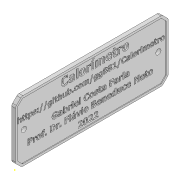
# Autodesk Inventor part: Placa
Saved by Autodesk Inventor 2020 (Build 240168000, 168)
## iProperties
Created: 2022-08-02
Part Number: Placa
Material: Genérico
Document SubType Name: Modeling
Designer: gabri
Density: 1 g/cm^3
Appearance: Padrão
Author: gabri
Autodesk Inventor part; units mm, degrees
(part 1 of 4)
ref_plane "YZ Plane" through (0, 0, 0) normal (1, 0, 0) x (0, 1, 0)
ref_plane "XZ Plane" through (0, 0, 0) normal (0, 1, 0) x (-1, 0, 0)
ref_plane "XY Plane" through (0, 0, 0) normal (0, 0, 1) x (1, 0, 0)
sketch "Esboço1" plane through (0, 0, 0) normal (1, 0, 0) x (0, 1, 0)
  line L0 (0, 0) -> (40, 0)
  line L1 (40, 0) -> (40, -100)
  line L2 (40, -100) -> (0, -100)
  line L3 (0, -100) -> (0, 0)
  dimension "d0" = 100
  dimension "d1" = 40
  constraints: 8 end point, 2 parallel, 1 horizontal, 1 perpendicular
  measures "d0" distance of L2.end L0.start
  measures "d1" distance of L1.end L2.end
extrude "Extrusão1" add sketch "Esboço1" along normal blind 2
sketch "Esboço3" plane through (2, 0, 0) normal (1, 0, 0) x (0, 0, -1)
  circle A0 centre (94, 20) radius 1.75
  circle A1 centre (6, 20) radius 1.75
  line L0 (100, 0) -> (100, 40) projected
  line L1 (0, 40) -> (0, 0) projected
  line L2 (0, 0) -> (100, 0) projected
  dimension "d4" = 3.5
  dimension "d5" = 3.5
  dimension "d6" = 6
  dimension "d7" = 6
  dimension "d10" = 40
  dimension "d11" = 20
  dimension "d12" = 20
  constraints: 2 centre point
  measures "d4" diameter of A0
  measures "d5" diameter of A1
  measures "d6" distance from line of L0 A0.centre
  measures "d7" distance from line of L1 A1.centre
  measures "d10" distance of L1.start L1.end
  measures "d11" distance from line of L2 A1.centre
  measures "d12" distance from line of L2 A0.centre
extrude "Extrusão2" cut sketch "Esboço3" against normal blind 4
sketch "Esboço2" plane through (2, 0, 0) normal (1, 0, 0) x (0, 0, -1)
  line L0 (30.0469, 37.5277) -> (51.3829, 37.5277) construction
  line L1 (51.3829, 37.5277) -> (51.3829, 32.8173) construction
  line L2 (51.3829, 32.8173) -> (30.0469, 32.8173) construction
  line L3 (30.0469, 32.8173) -> (30.0469, 37.5277) construction
  line L4 (1.6337, 28.6211) -> (100.4753, 28.6211) construction
  line L5 (100.4753, 28.6211) -> (100.4753, 23.9424) construction
  line L6 (100.4753, 23.9424) -> (1.6337, 23.9424) construction
  line L7 (1.6337, 23.9424) -> (1.6337, 28.6211) construction
  line L8 (1.8628, 19.959) -> (97.4553, 19.959) construction
  line L9 (97.4553, 19.959) -> (97.4553, 12.3141) construction
  line L10 (97.4553, 12.3141) -> (1.8628, 12.3141) construction
  line L11 (1.8628, 12.3141) -> (1.8628, 19.959) construction
  line L12 (1.4175, 13.8251) -> (97.3864, 13.8251) construction
  line L13 (97.3864, 13.8251) -> (97.3864, 4.9391) construction
  line L14 (97.3864, 4.9391) -> (1.4175, 4.9391) construction
  line L15 (1.4175, 4.9391) -> (1.4175, 13.8251) construction
  line L16 (0.4004, 6.6404) -> (95.5795, 6.6404) construction
  line L17 (95.5795, 6.6404) -> (95.5795, -2.443) construction
  line L18 (95.5795, -2.443) -> (0.4004, -2.443) construction
  line L19 (0.4004, -2.443) -> (0.4004, 6.6404) construction
  spline S0 degree 2 poles (32.9886, 31.2299) (31.7495, 31.2299) (30.2965, 32.7275) (30.2965, 34.0824) knots 0 0 0 1 2 2 2
  spline S1 degree 2 poles (30.2965, 34.0824) (30.2965, 35.3883) (31.7539, 36.9438) (32.993, 36.9438) knots 0 0 0 1 2 2 2
  spline S2 degree 2 poles (32.993, 36.9438) (33.3184, 36.9438) (33.8443, 36.8681) (34.085, 36.8057) knots 0 0 0 1 2 2 2
  spline S3 degree 2 poles (34.085, 36.8057) (34.2722, 36.7477) (34.7134, 36.5561) (34.8516, 36.4848) knots 0 0 0 1 2 2 2
  line L20 (34.8516, 36.4848) -> (34.8516, 35.1744)
  line L21 (34.8516, 35.1744) -> (34.7134, 35.1744)
  spline S4 degree 2 poles (34.7134, 35.1744) (34.6109, 35.2635) (34.3078, 35.5131) (34.1162, 35.629) knots 0 0 0 1 2 2 2
  spline S5 degree 2 poles (34.1162, 35.629) (33.9245, 35.7493) (33.4655, 35.9143) (33.2114, 35.9143) knots 0 0 0 1 2 2 2
  spline S6 degree 2 poles (33.2114, 35.9143) (32.9128, 35.9143) (32.418, 35.7271) (32.1907, 35.4908) knots 0 0 0 1 2 2 2
  spline S7 degree 2 poles (32.1907, 35.4908) (31.9857, 35.2814) (31.7227, 34.5638) (31.7227, 34.078) knots 0 0 0 1 2 2 2
  spline S8 degree 2 poles (31.7227, 34.078) (31.7227, 33.5654) (31.9946, 32.8656) (32.2175, 32.6517) knots 0 0 0 1 2 2 2
  spline S9 degree 2 poles (32.2175, 32.6517) (32.4314, 32.4422) (32.9574, 32.2595) (33.2203, 32.2595) knots 0 0 0 1 2 2 2
  spline S10 degree 2 poles (33.2203, 32.2595) (33.4922, 32.2595) (33.9869, 32.4422) (34.1563, 32.5536) knots 0 0 0 1 2 2 2
  spline S11 degree 2 poles (34.1563, 32.5536) (34.3435, 32.6651) (34.6243, 32.9013) (34.7268, 32.9949) knots 0 0 0 1 2 2 2
  line L22 (34.7268, 32.9949) -> (34.8516, 32.9949)
  line L23 (34.8516, 32.9949) -> (34.8516, 31.7023)
  spline S12 degree 2 poles (34.8516, 31.7023) (34.7001, 31.631) (34.3034, 31.4528) (34.0894, 31.3904) knots 0 0 0 1 2 2 2
  spline S13 degree 2 poles (34.0894, 31.3904) (33.8309, 31.3101) (33.3808, 31.2299) (32.9886, 31.2299) knots 0 0 0 1 2 2 2
  spline S14 degree 2 poles (37.8779, 31.7781) (37.7442, 31.6667) (37.5347, 31.4884) (37.3565, 31.3993) knots 0 0 0 1 2 2 2
  spline S15 degree 2 poles (37.3565, 31.3993) (37.1826, 31.3146) (36.8528, 31.2254) (36.5586, 31.2254) knots 0 0 0 1 2 2 2
  spline S16 degree 2 poles (36.5586, 31.2254) (36.006, 31.2254) (35.2795, 31.9653) (35.2795, 32.5269) knots 0 0 0 1 2 2 2
  spline S17 degree 2 poles (35.2795, 32.5269) (35.2795, 32.986) (35.6494, 33.5565) (35.9971, 33.7214) knots 0 0 0 1 2 2 2
  spline S18 degree 2 poles (35.9971, 33.7214) (36.3492, 33.8908) (37.3253, 34.0245) (37.8869, 34.0601) knots 0 0 0 1 2 2 2
  line L24 (37.8869, 34.0601) -> (37.8869, 34.0824)
  spline S19 degree 2 poles (37.8869, 34.0824) (37.8869, 34.4256) (37.3787, 34.6886) (36.8706, 34.6886) knots 0 0 0 1 2 2 2
  spline S20 degree 2 poles (36.8706, 34.6886) (36.6433, 34.6886) (36.0283, 34.5237) (35.7386, 34.3944) knots 0 0 0 1 2 2 2
  line L25 (35.7386, 34.3944) -> (35.6271, 34.3944)
  line L26 (35.6271, 34.3944) -> (35.6271, 35.3972)
  spline S21 degree 2 poles (35.6271, 35.3972) (35.8188, 35.4507) (36.6745, 35.6023) (37.1113, 35.6023) knots 0 0 0 1 2 2 2
  spline S22 degree 2 poles (37.1113, 35.6023) (38.181, 35.6023) (39.1616, 34.8891) (39.1616, 34.1582) knots 0 0 0 1 2 2 2
  line L27 (39.1616, 34.1582) -> (39.1616, 31.3369)
  line L28 (39.1616, 31.3369) -> (37.8779, 31.3369)
  line L29 (37.8779, 31.3369) -> (37.8779, 31.7781)
  line L30 (37.8779, 32.4199) -> (37.8779, 33.2801)
  spline S23 degree 2 poles (37.8779, 33.2801) (37.5481, 33.2489) (37.1425, 33.1999) (36.9464, 33.1286) knots 0 0 0 1 2 2 2
  spline S24 degree 2 poles (36.9464, 33.1286) (36.7726, 33.0707) (36.5854, 32.83) (36.5854, 32.6339) knots 0 0 0 1 2 2 2
  spline S25 degree 2 poles (36.5854, 32.6339) (36.5854, 32.3442) (36.9018, 32.1258) (37.2094, 32.1258) knots 0 0 0 1 2 2 2
  spline S26 degree 2 poles (37.2094, 32.1258) (37.3787, 32.1258) (37.7353, 32.2818) (37.8779, 32.4199) knots 0 0 0 1 2 2 2
  line L31 (41.4124, 31.3369) -> (40.1198, 31.3369)
  line L32 (40.1198, 31.3369) -> (40.1198, 37.082)
  line L33 (40.1198, 37.082) -> (41.4124, 37.082)
  line L34 (41.4124, 37.082) -> (41.4124, 31.3369)
  spline S27 degree 2 poles (46.382, 33.4094) (46.382, 32.3843) (45.2633, 31.2076) (44.2426, 31.2076) knots 0 0 0 1 2 2 2
  spline S28 degree 2 poles (44.2426, 31.2076) (43.2264, 31.2076) (42.0988, 32.3843) (42.0988, 33.4094) knots 0 0 0 1 2 2 2
  spline S29 degree 2 poles (42.0988, 33.4094) (42.0988, 34.4434) (43.2264, 35.6156) (44.2426, 35.6156) knots 0 0 0 1 2 2 2
  spline S30 degree 2 poles (44.2426, 35.6156) (45.2588, 35.6156) (46.382, 34.439) (46.382, 33.4094) knots 0 0 0 1 2 2 2
  spline S31 degree 2 poles (45.0582, 33.4005) (45.0582, 33.7704) (44.9379, 34.2651) (44.8309, 34.4122) knots 0 0 0 1 2 2 2
  spline S32 degree 2 poles (44.8309, 34.4122) (44.7151, 34.5682) (44.4253, 34.6886) (44.2426, 34.6886) knots 0 0 0 1 2 2 2
  spline S33 degree 2 poles (44.2426, 34.6886) (44.0643, 34.6886) (43.7835, 34.5816) (43.6676, 34.4301) knots 0 0 0 1 2 2 2
  spline S34 degree 2 poles (43.6676, 34.4301) (43.5562, 34.2874) (43.4225, 33.7838) (43.4225, 33.4005) knots 0 0 0 1 2 2 2
  spline S35 degree 2 poles (43.4225, 33.4005) (43.4225, 33.0216) (43.5473, 32.5536) (43.6498, 32.411) knots 0 0 0 1 2 2 2
  spline S36 degree 2 poles (43.6498, 32.411) (43.7523, 32.2684) (44.0643, 32.1347) (44.2515, 32.1347) knots 0 0 0 1 2 2 2
  spline S37 degree 2 poles (44.2515, 32.1347) (44.4075, 32.1347) (44.7284, 32.2684) (44.8265, 32.4021) knots 0 0 0 1 2 2 2
  spline S38 degree 2 poles (44.8265, 32.4021) (44.9379, 32.5581) (45.0582, 33.0083) (45.0582, 33.4005) knots 0 0 0 1 2 2 2
  line L35 (49.854, 34.2607) -> (49.7471, 34.2607)
  spline S39 degree 2 poles (49.7471, 34.2607) (49.6713, 34.2874) (49.3905, 34.3142) (49.2211, 34.3142) knots 0 0 0 1 2 2 2
  spline S40 degree 2 poles (49.2211, 34.3142) (49.0206, 34.3142) (48.5704, 34.1938) (48.3609, 34.1136) knots 0 0 0 1 2 2 2
  line L36 (48.3609, 34.1136) -> (48.3609, 31.3369)
  line L37 (48.3609, 31.3369) -> (47.0684, 31.3369)
  line L38 (47.0684, 31.3369) -> (47.0684, 35.4864)
  line L39 (47.0684, 35.4864) -> (48.3609, 35.4864)
  line L40 (48.3609, 35.4864) -> (48.3609, 34.8891)
  spline S41 degree 2 poles (48.3609, 34.8891) (48.4501, 34.9694) (48.7621, 35.219) (48.8913, 35.2947) knots 0 0 0 1 2 2 2
  spline S42 degree 2 poles (48.8913, 35.2947) (49.0339, 35.3794) (49.4083, 35.4998) (49.5732, 35.4998) knots 0 0 0 1 2 2 2
  spline S43 degree 2 poles (49.5732, 35.4998) (49.6356, 35.4998) (49.7916, 35.4908) (49.854, 35.4864) knots 0 0 0 1 2 2 2
  line L41 (49.854, 35.4864) -> (49.854, 34.2607)
  line L42 (51.6413, 31.3369) -> (50.3488, 31.3369)
  line L43 (50.3488, 31.3369) -> (50.3488, 35.4864)
  line L44 (50.3488, 35.4864) -> (51.6413, 35.4864)
  line L45 (51.6413, 35.4864) -> (51.6413, 31.3369)
  line L46 (52.194, 37.5277) -> (51.0842, 36.0747)
  line L47 (51.0842, 36.0747) -> (50.2061, 36.0747)
  line L48 (50.2061, 36.0747) -> (50.9728, 37.5277)
  line L49 (50.9728, 37.5277) -> (52.194, 37.5277)
  line L50 (57.5826, 31.3369) -> (57.5826, 33.4094)
  spline S44 degree 2 poles (57.5826, 33.4094) (57.5826, 33.7169) (57.5603, 34.1359) (57.5068, 34.2696) knots 0 0 0 1 2 2 2
  spline S45 degree 2 poles (57.5068, 34.2696) (57.4488, 34.4033) (57.2171, 34.5237) (57.0076, 34.5237) knots 0 0 0 1 2 2 2
  spline S46 degree 2 poles (57.0076, 34.5237) (56.8605, 34.5237) (56.5753, 34.3944) (56.4059, 34.2741) knots 0 0 0 1 2 2 2
  line L51 (56.4059, 34.2741) -> (56.4059, 31.3369)
  line L52 (56.4059, 31.3369) -> (55.1044, 31.3369)
  line L53 (55.1044, 31.3369) -> (55.1044, 33.4094)
  spline S47 degree 2 poles (55.1044, 33.4094) (55.1044, 33.7125) (55.0777, 34.1359) (55.0242, 34.2696) knots 0 0 0 1 2 2 2
  spline S48 degree 2 poles (55.0242, 34.2696) (54.9663, 34.4033) (54.7345, 34.5237) (54.525, 34.5237) knots 0 0 0 1 2 2 2
  spline S49 degree 2 poles (54.525, 34.5237) (54.369, 34.5237) (54.0615, 34.3766) (53.9189, 34.2741) knots 0 0 0 1 2 2 2
  line L54 (53.9189, 34.2741) -> (53.9189, 31.3369)
  line L55 (53.9189, 31.3369) -> (52.6263, 31.3369)
  line L56 (52.6263, 31.3369) -> (52.6263, 35.4864)
  line L57 (52.6263, 35.4864) -> (53.9189, 35.4864)
  line L58 (53.9189, 35.4864) -> (53.9189, 35.0273)
  spline S50 degree 2 poles (53.9189, 35.0273) (54.2353, 35.2947) (54.8014, 35.5978) (55.1535, 35.5978) knots 0 0 0 1 2 2 2
  spline S51 degree 2 poles (55.1535, 35.5978) (55.5323, 35.5978) (56.1117, 35.2368) (56.2633, 34.8758) knots 0 0 0 1 2 2 2
  spline S52 degree 2 poles (56.2633, 34.8758) (56.6332, 35.2234) (57.2928, 35.5978) (57.6316, 35.5978) knots 0 0 0 1 2 2 2
  spline S53 degree 2 poles (57.6316, 35.5978) (57.9213, 35.5978) (58.3804, 35.4151) (58.5364, 35.2279) knots 0 0 0 1 2 2 2
  spline S54 degree 2 poles (58.5364, 35.2279) (58.7102, 35.0273) (58.884, 34.4791) (58.884, 34.0378) knots 0 0 0 1 2 2 2
  line L59 (58.884, 34.0378) -> (58.884, 31.3369)
  line L60 (58.884, 31.3369) -> (57.5826, 31.3369)
  spline S55 degree 2 poles (61.9683, 31.2254) (60.7916, 31.2254) (59.5392, 32.3486) (59.5392, 33.3871) knots 0 0 0 1 2 2 2
  spline S56 degree 2 poles (59.5392, 33.3871) (59.5392, 34.4033) (60.7069, 35.6156) (61.7588, 35.6156) knots 0 0 0 1 2 2 2
  spline S57 degree 2 poles (61.7588, 35.6156) (62.7082, 35.6156) (63.6709, 34.5861) (63.6709, 33.6322) knots 0 0 0 1 2 2 2
  line L61 (63.6709, 33.6322) -> (63.6709, 33.1643)
  line L62 (63.6709, 33.1643) -> (60.8317, 33.1643)
  spline S58 degree 2 poles (60.8317, 33.1643) (60.8496, 32.8745) (61.0591, 32.4912) (61.2284, 32.3754) knots 0 0 0 1 2 2 2
  spline S59 degree 2 poles (61.2284, 32.3754) (61.3933, 32.2595) (61.839, 32.1614) (62.102, 32.1614) knots 0 0 0 1 2 2 2
  spline S60 degree 2 poles (62.102, 32.1614) (62.3249, 32.1614) (62.7616, 32.2595) (62.9444, 32.3442) knots 0 0 0 1 2 2 2
  spline S61 degree 2 poles (62.9444, 32.3442) (63.1048, 32.411) (63.3723, 32.5759) (63.4569, 32.6383) knots 0 0 0 1 2 2 2
  line L63 (63.4569, 32.6383) -> (63.5951, 32.6383)
  line L64 (63.5951, 32.6383) -> (63.5951, 31.5686)
  spline S62 degree 2 poles (63.5951, 31.5686) (63.4347, 31.5062) (63.1762, 31.3993) (62.9444, 31.3458) knots 0 0 0 1 2 2 2
  spline S63 degree 2 poles (62.9444, 31.3458) (62.7349, 31.2878) (62.2892, 31.2254) (61.9683, 31.2254) knots 0 0 0 1 2 2 2
  spline S64 degree 2 poles (62.3962, 33.9442) (62.3873, 34.3543) (62.0262, 34.7866) (61.6563, 34.7866) knots 0 0 0 1 2 2 2
  spline S65 degree 2 poles (61.6563, 34.7866) (61.2775, 34.7866) (60.8496, 34.332) (60.8273, 33.9442) knots 0 0 0 1 2 2 2
  line L65 (60.8273, 33.9442) -> (62.3962, 33.9442)
  spline S66 degree 2 poles (65.9217, 31.2566) (65.1328, 31.2566) (64.4108, 31.9074) (64.4108, 32.6472) knots 0 0 0 1 2 2 2
  line L66 (64.4108, 32.6472) -> (64.4108, 34.5861)
  line L67 (64.4108, 34.5861) -> (63.916, 34.5861)
  line L68 (63.916, 34.5861) -> (63.916, 35.4864)
  line L69 (63.916, 35.4864) -> (64.4108, 35.4864)
  line L70 (64.4108, 35.4864) -> (64.4108, 36.672)
  line L71 (64.4108, 36.672) -> (65.7033, 36.672)
  line L72 (65.7033, 36.672) -> (65.7033, 35.4864)
  line L73 (65.7033, 35.4864) -> (66.9513, 35.4864)
  line L74 (66.9513, 35.4864) -> (66.9513, 34.5861)
  line L75 (66.9513, 34.5861) -> (65.7033, 34.5861)
  line L76 (65.7033, 34.5861) -> (65.7033, 33.1108)
  spline S67 degree 2 poles (65.7033, 33.1108) (65.7033, 32.8924) (65.7122, 32.567) (65.7657, 32.4378) knots 0 0 0 1 2 2 2
  spline S68 degree 2 poles (65.7657, 32.4378) (65.8192, 32.3085) (66.0822, 32.157) (66.3317, 32.157) knots 0 0 0 1 2 2 2
  spline S69 degree 2 poles (66.3317, 32.157) (66.4387, 32.157) (66.773, 32.2461) (66.8398, 32.2818) knots 0 0 0 1 2 2 2
  line L77 (66.8398, 32.2818) -> (66.9513, 32.2818)
  line L78 (66.9513, 32.2818) -> (66.9513, 31.3725)
  spline S70 degree 2 poles (66.9513, 31.3725) (66.7418, 31.319) (66.2693, 31.2566) (65.9217, 31.2566) knots 0 0 0 1 2 2 2
  line L79 (70.2629, 34.2607) -> (70.1559, 34.2607)
  spline S71 degree 2 poles (70.1559, 34.2607) (70.0801, 34.2874) (69.7993, 34.3142) (69.63, 34.3142) knots 0 0 0 1 2 2 2
  spline S72 degree 2 poles (69.63, 34.3142) (69.4294, 34.3142) (68.9792, 34.1938) (68.7698, 34.1136) knots 0 0 0 1 2 2 2
  line L80 (68.7698, 34.1136) -> (68.7698, 31.3369)
  line L81 (68.7698, 31.3369) -> (67.4772, 31.3369)
  line L82 (67.4772, 31.3369) -> (67.4772, 35.4864)
  line L83 (67.4772, 35.4864) -> (68.7698, 35.4864)
  line L84 (68.7698, 35.4864) -> (68.7698, 34.8891)
  spline S73 degree 2 poles (68.7698, 34.8891) (68.8589, 34.9694) (69.1709, 35.219) (69.3001, 35.2947) knots 0 0 0 1 2 2 2
  spline S74 degree 2 poles (69.3001, 35.2947) (69.4428, 35.3794) (69.8172, 35.4998) (69.9821, 35.4998) knots 0 0 0 1 2 2 2
  spline S75 degree 2 poles (69.9821, 35.4998) (70.0445, 35.4998) (70.2005, 35.4908) (70.2629, 35.4864) knots 0 0 0 1 2 2 2
  line L85 (70.2629, 35.4864) -> (70.2629, 34.2607)
  spline S76 degree 2 poles (74.7377, 33.4094) (74.7377, 32.3843) (73.619, 31.2076) (72.5984, 31.2076) knots 0 0 0 1 2 2 2
  spline S77 degree 2 poles (72.5984, 31.2076) (71.5822, 31.2076) (70.4545, 32.3843) (70.4545, 33.4094) knots 0 0 0 1 2 2 2
  spline S78 degree 2 poles (70.4545, 33.4094) (70.4545, 34.4434) (71.5822, 35.6156) (72.5984, 35.6156) knots 0 0 0 1 2 2 2
  spline S79 degree 2 poles (72.5984, 35.6156) (73.6146, 35.6156) (74.7377, 34.439) (74.7377, 33.4094) knots 0 0 0 1 2 2 2
  spline S80 degree 2 poles (73.414, 33.4005) (73.414, 33.7704) (73.2937, 34.2651) (73.1867, 34.4122) knots 0 0 0 1 2 2 2
  spline S81 degree 2 poles (73.1867, 34.4122) (73.0708, 34.5682) (72.7811, 34.6886) (72.5984, 34.6886) knots 0 0 0 1 2 2 2
  spline S82 degree 2 poles (72.5984, 34.6886) (72.4201, 34.6886) (72.1393, 34.5816) (72.0234, 34.4301) knots 0 0 0 1 2 2 2
  spline S83 degree 2 poles (72.0234, 34.4301) (71.912, 34.2874) (71.7783, 33.7838) (71.7783, 33.4005) knots 0 0 0 1 2 2 2
  spline S84 degree 2 poles (71.7783, 33.4005) (71.7783, 33.0216) (71.9031, 32.5536) (72.0056, 32.411) knots 0 0 0 1 2 2 2
  spline S85 degree 2 poles (72.0056, 32.411) (72.1081, 32.2684) (72.4201, 32.1347) (72.6073, 32.1347) knots 0 0 0 1 2 2 2
  spline S86 degree 2 poles (72.6073, 32.1347) (72.7633, 32.1347) (73.0842, 32.2684) (73.1822, 32.4021) knots 0 0 0 1 2 2 2
  spline S87 degree 2 poles (73.1822, 32.4021) (73.2937, 32.5581) (73.414, 33.0083) (73.414, 33.4005) knots 0 0 0 1 2 2 2
  line L86 (4.4189, 24.9623) -> (3.5907, 24.9623)
  line L87 (3.5907, 24.9623) -> (3.5907, 26.2698)
  spline S88 degree 2 poles (3.5907, 26.2698) (3.5907, 26.4315) (3.5652, 26.7491) (3.5312, 26.8229) knots 0 0 0 1 2 2 2
  spline S89 degree 2 poles (3.5312, 26.8229) (3.4886, 26.9136) (3.3298, 26.9902) (3.1936, 26.9902) knots 0 0 0 1 2 2 2
  spline S90 degree 2 poles (3.1936, 26.9902) (3.0944, 26.9902) (2.8873, 26.9136) (2.771, 26.8314) knots 0 0 0 1 2 2 2
  line L88 (2.771, 26.8314) -> (2.771, 24.9623)
  line L89 (2.771, 24.9623) -> (1.9485, 24.9623)
  line L90 (1.9485, 24.9623) -> (1.9485, 28.6183)
  line L91 (1.9485, 28.6183) -> (2.771, 28.6183)
  line L92 (2.771, 28.6183) -> (2.771, 27.3107)
  spline S91 degree 2 poles (2.771, 27.3107) (2.9724, 27.4809) (3.3553, 27.6738) (3.5879, 27.6738) knots 0 0 0 1 2 2 2
  spline S92 degree 2 poles (3.5879, 27.6738) (3.9906, 27.6738) (4.4189, 27.1632) (4.4189, 26.6811) knots 0 0 0 1 2 2 2
  line L93 (4.4189, 26.6811) -> (4.4189, 24.9623)
  spline S93 degree 2 poles (6.0385, 24.9112) (5.5364, 24.9112) (5.0769, 25.3253) (5.0769, 25.7961) knots 0 0 0 1 2 2 2
  line L94 (5.0769, 25.7961) -> (5.0769, 27.0299)
  line L95 (5.0769, 27.0299) -> (4.7621, 27.0299)
  line L96 (4.7621, 27.0299) -> (4.7621, 27.6029)
  line L97 (4.7621, 27.6029) -> (5.0769, 27.6029)
  line L98 (5.0769, 27.6029) -> (5.0769, 28.3573)
  line L99 (5.0769, 28.3573) -> (5.8995, 28.3573)
  line L100 (5.8995, 28.3573) -> (5.8995, 27.6029)
  line L101 (5.8995, 27.6029) -> (6.6936, 27.6029)
  line L102 (6.6936, 27.6029) -> (6.6936, 27.0299)
  line L103 (6.6936, 27.0299) -> (5.8995, 27.0299)
  line L104 (5.8995, 27.0299) -> (5.8995, 26.0911)
  spline S94 degree 2 poles (5.8995, 26.0911) (5.8995, 25.9521) (5.9051, 25.7451) (5.9392, 25.6628) knots 0 0 0 1 2 2 2
  spline S95 degree 2 poles (5.9392, 25.6628) (5.9732, 25.5806) (6.1406, 25.4841) (6.2994, 25.4841) knots 0 0 0 1 2 2 2
  spline S96 degree 2 poles (6.2994, 25.4841) (6.3675, 25.4841) (6.5802, 25.5409) (6.6227, 25.5636) knots 0 0 0 1 2 2 2
  line L105 (6.6227, 25.5636) -> (6.6936, 25.5636)
  line L106 (6.6936, 25.5636) -> (6.6936, 24.985)
  spline S97 degree 2 poles (6.6936, 24.985) (6.5603, 24.9509) (6.2597, 24.9112) (6.0385, 24.9112) knots 0 0 0 1 2 2 2
  spline S98 degree 2 poles (8.0381, 24.9112) (7.536, 24.9112) (7.0765, 25.3253) (7.0765, 25.7961) knots 0 0 0 1 2 2 2
  line L107 (7.0765, 25.7961) -> (7.0765, 27.0299)
  line L108 (7.0765, 27.0299) -> (6.7617, 27.0299)
  line L109 (6.7617, 27.0299) -> (6.7617, 27.6029)
  line L110 (6.7617, 27.6029) -> (7.0765, 27.6029)
  line L111 (7.0765, 27.6029) -> (7.0765, 28.3573)
  line L112 (7.0765, 28.3573) -> (7.8991, 28.3573)
  line L113 (7.8991, 28.3573) -> (7.8991, 27.6029)
  line L114 (7.8991, 27.6029) -> (8.6932, 27.6029)
  line L115 (8.6932, 27.6029) -> (8.6932, 27.0299)
  line L116 (8.6932, 27.0299) -> (7.8991, 27.0299)
  line L117 (7.8991, 27.0299) -> (7.8991, 26.0911)
  spline S99 degree 2 poles (7.8991, 26.0911) (7.8991, 25.9521) (7.9047, 25.7451) (7.9388, 25.6628) knots 0 0 0 1 2 2 2
  spline S100 degree 2 poles (7.9388, 25.6628) (7.9728, 25.5806) (8.1402, 25.4841) (8.299, 25.4841) knots 0 0 0 1 2 2 2
  spline S101 degree 2 poles (8.299, 25.4841) (8.3671, 25.4841) (8.5798, 25.5409) (8.6223, 25.5636) knots 0 0 0 1 2 2 2
  line L118 (8.6223, 25.5636) -> (8.6932, 25.5636)
  line L119 (8.6932, 25.5636) -> (8.6932, 24.985)
  spline S102 degree 2 poles (8.6932, 24.985) (8.5599, 24.9509) (8.2593, 24.9112) (8.0381, 24.9112) knots 0 0 0 1 2 2 2
  spline S103 degree 2 poles (11.6146, 26.318) (11.6146, 25.6855) (10.9736, 24.9112) (10.5028, 24.9112) knots 0 0 0 1 2 2 2
  spline S104 degree 2 poles (10.5028, 24.9112) (10.3071, 24.9112) (10.015, 24.9991) (9.8504, 25.0956) knots 0 0 0 1 2 2 2
  line L120 (9.8504, 25.0956) -> (9.8504, 23.9951)
  line L121 (9.8504, 23.9951) -> (9.0279, 23.9951)
  line L122 (9.0279, 23.9951) -> (9.0279, 27.6029)
  line L123 (9.0279, 27.6029) -> (9.8504, 27.6029)
  line L124 (9.8504, 27.6029) -> (9.8504, 27.3249)
  spline S105 degree 2 poles (9.8504, 27.3249) (10.032, 27.4809) (10.4064, 27.6738) (10.6531, 27.6738) knots 0 0 0 1 2 2 2
  spline S106 degree 2 poles (10.6531, 27.6738) (11.1126, 27.6738) (11.6146, 26.9448) (11.6146, 26.318) knots 0 0 0 1 2 2 2
  spline S107 degree 2 poles (10.7722, 26.301) (10.7722, 26.6867) (10.534, 27.0328) (10.2844, 27.0328) knots 0 0 0 1 2 2 2
  spline S108 degree 2 poles (10.2844, 27.0328) (10.1738, 27.0328) (9.9554, 26.9619) (9.8504, 26.8909) knots 0 0 0 1 2 2 2
  line L125 (9.8504, 26.8909) -> (9.8504, 25.5664)
  spline S109 degree 2 poles (9.8504, 25.5664) (9.9157, 25.538) (10.0745, 25.5153) (10.1823, 25.5153) knots 0 0 0 1 2 2 2
  spline S110 degree 2 poles (10.1823, 25.5153) (10.4801, 25.5153) (10.7722, 25.9068) (10.7722, 26.301) knots 0 0 0 1 2 2 2
  spline S111 degree 2 poles (12.8598, 24.8914) (12.5705, 24.8914) (12.0514, 25.019) (11.8812, 25.1041) knots 0 0 0 1 2 2 2
  line L126 (11.8812, 25.1041) -> (11.8812, 25.799)
  line L127 (11.8812, 25.799) -> (11.9493, 25.799)
  spline S112 degree 2 poles (11.9493, 25.799) (12.0089, 25.7536) (12.1592, 25.6458) (12.2925, 25.5862) knots 0 0 0 1 2 2 2
  spline S113 degree 2 poles (12.2925, 25.5862) (12.4088, 25.5324) (12.6953, 25.4558) (12.8654, 25.4558) knots 0 0 0 1 2 2 2
  spline S114 degree 2 poles (12.8654, 25.4558) (13.0385, 25.4558) (13.3051, 25.5636) (13.3051, 25.6798) knots 0 0 0 1 2 2 2
  spline S115 degree 2 poles (13.3051, 25.6798) (13.3051, 25.7706) (13.1831, 25.867) (13.0073, 25.9068) knots 0 0 0 1 2 2 2
  spline S116 degree 2 poles (13.0073, 25.9068) (12.9137, 25.9323) (12.6272, 25.9862) (12.5166, 26.0202) knots 0 0 0 1 2 2 2
  spline S117 degree 2 poles (12.5166, 26.0202) (12.2046, 26.1166) (11.8926, 26.4939) (11.8926, 26.803) knots 0 0 0 1 2 2 2
  spline S118 degree 2 poles (11.8926, 26.803) (11.8926, 26.9789) (12.0543, 27.2909) (12.2131, 27.4128) knots 0 0 0 1 2 2 2
  spline S119 degree 2 poles (12.2131, 27.4128) (12.3691, 27.532) (12.8314, 27.6738) (13.1235, 27.6738) knots 0 0 0 1 2 2 2
  spline S120 degree 2 poles (13.1235, 27.6738) (13.4015, 27.6738) (13.8667, 27.5632) (14.0255, 27.4866) knots 0 0 0 1 2 2 2
  line L128 (14.0255, 27.4866) -> (14.0255, 26.8172)
  line L129 (14.0255, 26.8172) -> (13.9603, 26.8172)
  spline S121 degree 2 poles (13.9603, 26.8172) (13.9177, 26.8512) (13.7334, 26.9619) (13.6483, 27.0016) knots 0 0 0 1 2 2 2
  spline S122 degree 2 poles (13.6483, 27.0016) (13.5433, 27.0469) (13.2881, 27.1093) (13.1547, 27.1093) knots 0 0 0 1 2 2 2
  spline S123 degree 2 poles (13.1547, 27.1093) (12.9761, 27.1093) (12.7293, 26.9874) (12.7293, 26.8881) knots 0 0 0 1 2 2 2
  spline S124 degree 2 poles (12.7293, 26.8881) (12.7293, 26.7974) (12.8513, 26.6952) (13.0555, 26.6442) knots 0 0 0 1 2 2 2
  spline S125 degree 2 poles (13.0555, 26.6442) (13.1604, 26.6187) (13.4355, 26.5704) (13.5632, 26.5279) knots 0 0 0 1 2 2 2
  spline S126 degree 2 poles (13.5632, 26.5279) (13.8468, 26.4371) (14.1418, 26.0826) (14.1418, 25.7876) knots 0 0 0 1 2 2 2
  spline S127 degree 2 poles (14.1418, 25.7876) (14.1418, 25.6033) (13.9688, 25.2657) (13.8071, 25.1523) knots 0 0 0 1 2 2 2
  spline S128 degree 2 poles (13.8071, 25.1523) (13.6398, 25.0275) (13.1803, 24.8914) (12.8598, 24.8914) knots 0 0 0 1 2 2 2
  line L130 (15.5089, 24.9623) -> (14.6778, 24.9623)
  line L131 (14.6778, 24.9623) -> (14.6778, 25.8869)
  line L132 (14.6778, 25.8869) -> (15.5089, 25.8869)
  line L133 (15.5089, 25.8869) -> (15.5089, 24.9623)
  line L134 (15.5089, 26.6782) -> (14.6778, 26.6782)
  line L135 (14.6778, 26.6782) -> (14.6778, 27.6029)
  line L136 (14.6778, 27.6029) -> (15.5089, 27.6029)
  line L137 (15.5089, 27.6029) -> (15.5089, 26.6782)
  line L138 (18.3111, 28.6183) -> (16.9185, 24.2021)
  line L139 (16.9185, 24.2021) -> (16.2435, 24.2021)
  line L140 (16.2435, 24.2021) -> (17.6333, 28.6183)
  line L141 (17.6333, 28.6183) -> (18.3111, 28.6183)
  line L142 (21.0879, 28.6183) -> (19.6953, 24.2021)
  line L143 (19.6953, 24.2021) -> (19.0202, 24.2021)
  line L144 (19.0202, 24.2021) -> (20.41, 28.6183)
  line L145 (20.41, 28.6183) -> (21.0879, 28.6183)
  spline S129 degree 2 poles (24.2334, 25.2657) (24.2334, 24.8999) (24.0206, 24.3865) (23.8391, 24.2447) knots 0 0 0 1 2 2 2
  spline S130 degree 2 poles (23.8391, 24.2447) (23.6547, 24.1) (23.1442, 23.9696) (22.8322, 23.9696) knots 0 0 0 1 2 2 2
  spline S131 degree 2 poles (22.8322, 23.9696) (22.5684, 23.9696) (22.0948, 24.0376) (21.9218, 24.083) knots 0 0 0 1 2 2 2
  line L146 (21.9218, 24.083) -> (21.9218, 24.7439)
  line L147 (21.9218, 24.7439) -> (22.0182, 24.7439)
  spline S132 degree 2 poles (22.0182, 24.7439) (22.0778, 24.7212) (22.2451, 24.6644) (22.3302, 24.6418) knots 0 0 0 1 2 2 2
  spline S133 degree 2 poles (22.3302, 24.6418) (22.4323, 24.6162) (22.6252, 24.5822) (22.7244, 24.5822) knots 0 0 0 1 2 2 2
  spline S134 degree 2 poles (22.7244, 24.5822) (22.9343, 24.5822) (23.2123, 24.6673) (23.2832, 24.7467) knots 0 0 0 1 2 2 2
  spline S135 degree 2 poles (23.2832, 24.7467) (23.3541, 24.829) (23.4108, 25.0502) (23.4108, 25.2204) knots 0 0 0 1 2 2 2
  line L148 (23.4108, 25.2204) -> (23.4108, 25.2686)
  spline S136 degree 2 poles (23.4108, 25.2686) (23.2718, 25.1466) (22.9088, 24.9991) (22.7159, 24.9991) knots 0 0 0 1 2 2 2
  spline S137 degree 2 poles (22.7159, 24.9991) (22.2026, 24.9991) (21.6466, 25.6657) (21.6466, 26.3492) knots 0 0 0 1 2 2 2
  spline S138 degree 2 poles (21.6466, 26.3492) (21.6466, 26.6584) (21.8168, 27.1519) (21.97, 27.3249) knots 0 0 0 1 2 2 2
  spline S139 degree 2 poles (21.97, 27.3249) (22.1175, 27.4922) (22.5287, 27.6738) (22.7528, 27.6738) knots 0 0 0 1 2 2 2
  spline S140 degree 2 poles (22.7528, 27.6738) (22.9542, 27.6738) (23.2747, 27.5717) (23.4051, 27.4866) knots 0 0 0 1 2 2 2
  line L149 (23.4051, 27.4866) -> (23.4363, 27.6029)
  line L150 (23.4363, 27.6029) -> (24.2334, 27.6029)
  line L151 (24.2334, 27.6029) -> (24.2334, 25.2657)
  line L152 (23.4108, 25.7933) -> (23.4108, 26.9902)
  spline S141 degree 2 poles (23.4108, 26.9902) (23.3513, 27.0186) (23.1726, 27.0555) (23.0818, 27.0555) knots 0 0 0 1 2 2 2
  spline S142 degree 2 poles (23.0818, 27.0555) (22.7868, 27.0555) (22.489, 26.6726) (22.489, 26.3294) knots 0 0 0 1 2 2 2
  spline S143 degree 2 poles (22.489, 26.3294) (22.489, 26.1592) (22.5344, 25.9209) (22.594, 25.8302) knots 0 0 0 1 2 2 2
  spline S144 degree 2 poles (22.594, 25.8302) (22.6535, 25.7394) (22.8436, 25.6486) (22.991, 25.6486) knots 0 0 0 1 2 2 2
  spline S145 degree 2 poles (22.991, 25.6486) (23.1017, 25.6486) (23.3144, 25.7252) (23.4108, 25.7933) knots 0 0 0 1 2 2 2
  line L153 (25.6855, 24.9623) -> (24.863, 24.9623)
  line L154 (24.863, 24.9623) -> (24.863, 27.6029)
  line L155 (24.863, 27.6029) -> (25.6855, 27.6029)
  line L156 (25.6855, 27.6029) -> (25.6855, 24.9623)
  line L157 (25.7111, 27.9801) -> (24.8403, 27.9801)
  line L158 (24.8403, 27.9801) -> (24.8403, 28.6211)
  line L159 (24.8403, 28.6211) -> (25.7111, 28.6211)
  line L160 (25.7111, 28.6211) -> (25.7111, 27.9801)
  spline S146 degree 2 poles (27.3249, 24.9112) (26.8229, 24.9112) (26.3634, 25.3253) (26.3634, 25.7961) knots 0 0 0 1 2 2 2
  line L161 (26.3634, 25.7961) -> (26.3634, 27.0299)
  line L162 (26.3634, 27.0299) -> (26.0486, 27.0299)
  line L163 (26.0486, 27.0299) -> (26.0486, 27.6029)
  line L164 (26.0486, 27.6029) -> (26.3634, 27.6029)
  line L165 (26.3634, 27.6029) -> (26.3634, 28.3573)
  line L166 (26.3634, 28.3573) -> (27.1859, 28.3573)
  line L167 (27.1859, 28.3573) -> (27.1859, 27.6029)
  line L168 (27.1859, 27.6029) -> (27.9801, 27.6029)
  line L169 (27.9801, 27.6029) -> (27.9801, 27.0299)
  line L170 (27.9801, 27.0299) -> (27.1859, 27.0299)
  line L171 (27.1859, 27.0299) -> (27.1859, 26.0911)
  spline S147 degree 2 poles (27.1859, 26.0911) (27.1859, 25.9521) (27.1916, 25.7451) (27.2257, 25.6628) knots 0 0 0 1 2 2 2
  spline S148 degree 2 poles (27.2257, 25.6628) (27.2597, 25.5806) (27.427, 25.4841) (27.5859, 25.4841) knots 0 0 0 1 2 2 2
  spline S149 degree 2 poles (27.5859, 25.4841) (27.6539, 25.4841) (27.8667, 25.5409) (27.9092, 25.5636) knots 0 0 0 1 2 2 2
  line L172 (27.9092, 25.5636) -> (27.9801, 25.5636)
  line L173 (27.9801, 25.5636) -> (27.9801, 24.985)
  spline S150 degree 2 poles (27.9801, 24.985) (27.8468, 24.9509) (27.5462, 24.9112) (27.3249, 24.9112) knots 0 0 0 1 2 2 2
  line L174 (30.7852, 24.9623) -> (29.957, 24.9623)
  line L175 (29.957, 24.9623) -> (29.957, 26.2698)
  spline S151 degree 2 poles (29.957, 26.2698) (29.957, 26.4315) (29.9315, 26.7491) (29.8975, 26.8229) knots 0 0 0 1 2 2 2
  spline S152 degree 2 poles (29.8975, 26.8229) (29.8549, 26.9136) (29.6961, 26.9902) (29.5599, 26.9902) knots 0 0 0 1 2 2 2
  spline S153 degree 2 poles (29.5599, 26.9902) (29.4607, 26.9902) (29.2536, 26.9136) (29.1373, 26.8314) knots 0 0 0 1 2 2 2
  line L176 (29.1373, 26.8314) -> (29.1373, 24.9623)
  line L177 (29.1373, 24.9623) -> (28.3148, 24.9623)
  line L178 (28.3148, 24.9623) -> (28.3148, 28.6183)
  line L179 (28.3148, 28.6183) -> (29.1373, 28.6183)
  line L180 (29.1373, 28.6183) -> (29.1373, 27.3107)
  spline S154 degree 2 poles (29.1373, 27.3107) (29.3387, 27.4809) (29.7216, 27.6738) (29.9542, 27.6738) knots 0 0 0 1 2 2 2
  spline S155 degree 2 poles (29.9542, 27.6738) (30.3569, 27.6738) (30.7852, 27.1632) (30.7852, 26.6811) knots 0 0 0 1 2 2 2
  line L181 (30.7852, 26.6811) -> (30.7852, 24.9623)
  line L182 (33.8456, 24.9623) -> (33.0231, 24.9623)
  line L183 (33.0231, 24.9623) -> (33.0231, 25.2544)
  spline S156 degree 2 poles (33.0231, 25.2544) (32.8103, 25.0757) (32.453, 24.8885) (32.2062, 24.8885) knots 0 0 0 1 2 2 2
  spline S157 degree 2 poles (32.2062, 24.8885) (31.8148, 24.8885) (31.3752, 25.3849) (31.3752, 25.8841) knots 0 0 0 1 2 2 2
  line L184 (31.3752, 25.8841) -> (31.3752, 27.6029)
  line L185 (31.3752, 27.6029) -> (32.2034, 27.6029)
  line L186 (32.2034, 27.6029) -> (32.2034, 26.2925)
  spline S158 degree 2 poles (32.2034, 26.2925) (32.2034, 26.0883) (32.2232, 25.8273) (32.2629, 25.7394) knots 0 0 0 1 2 2 2
  spline S159 degree 2 poles (32.2629, 25.7394) (32.3026, 25.6572) (32.4586, 25.5721) (32.6004, 25.5721) knots 0 0 0 1 2 2 2
  spline S160 degree 2 poles (32.6004, 25.5721) (32.6855, 25.5721) (32.9238, 25.6572) (33.0231, 25.7309) knots 0 0 0 1 2 2 2
  line L187 (33.0231, 25.7309) -> (33.0231, 27.6029)
  line L188 (33.0231, 27.6029) -> (33.8456, 27.6029)
  line L189 (33.8456, 27.6029) -> (33.8456, 24.9623)
  spline S161 degree 2 poles (37.062, 26.318) (37.062, 25.6884) (36.4238, 24.9112) (35.9501, 24.9112) knots 0 0 0 1 2 2 2
  spline S162 degree 2 poles (35.9501, 24.9112) (35.7544, 24.9112) (35.4623, 24.9991) (35.2978, 25.0927) knots 0 0 0 1 2 2 2
  line L190 (35.2978, 25.0927) -> (35.2637, 24.9623)
  line L191 (35.2637, 24.9623) -> (34.4752, 24.9623)
  line L192 (34.4752, 24.9623) -> (34.4752, 28.6183)
  line L193 (34.4752, 28.6183) -> (35.2978, 28.6183)
  line L194 (35.2978, 28.6183) -> (35.2978, 27.3249)
  spline S163 degree 2 poles (35.2978, 27.3249) (35.4793, 27.4809) (35.8537, 27.6738) (36.1004, 27.6738) knots 0 0 0 1 2 2 2
  spline S164 degree 2 poles (36.1004, 27.6738) (36.5628, 27.6738) (37.062, 26.9562) (37.062, 26.318) knots 0 0 0 1 2 2 2
  spline S165 degree 2 poles (36.2196, 26.301) (36.2196, 26.6952) (35.9813, 27.0328) (35.7317, 27.0328) knots 0 0 0 1 2 2 2
  spline S166 degree 2 poles (35.7317, 27.0328) (35.6211, 27.0328) (35.4027, 26.9619) (35.2978, 26.8909) knots 0 0 0 1 2 2 2
  line L195 (35.2978, 26.8909) -> (35.2978, 25.5692)
  spline S167 degree 2 poles (35.2978, 25.5692) (35.38, 25.5352) (35.5474, 25.5125) (35.6296, 25.5125) knots 0 0 0 1 2 2 2
  spline S168 degree 2 poles (35.6296, 25.5125) (35.9274, 25.5125) (36.2196, 25.9068) (36.2196, 26.301) knots 0 0 0 1 2 2 2
  line L196 (38.3667, 24.9623) -> (37.5356, 24.9623)
  line L197 (37.5356, 24.9623) -> (37.5356, 25.8869)
  line L198 (37.5356, 25.8869) -> (38.3667, 25.8869)
  line L199 (38.3667, 25.8869) -> (38.3667, 24.9623)
  spline S169 degree 2 poles (40.3124, 24.8914) (39.9862, 24.8914) (39.4445, 25.0559) (39.2431, 25.226) knots 0 0 0 1 2 2 2
  spline S170 degree 2 poles (39.2431, 25.226) (39.0474, 25.3991) (38.8261, 25.9181) (38.8261, 26.2698) knots 0 0 0 1 2 2 2
  spline S171 degree 2 poles (38.8261, 26.2698) (38.8261, 26.6499) (39.0644, 27.1803) (39.2714, 27.3504) knots 0 0 0 1 2 2 2
  spline S172 degree 2 poles (39.2714, 27.3504) (39.4671, 27.5149) (40.0004, 27.6738) (40.2897, 27.6738) knots 0 0 0 1 2 2 2
  spline S173 degree 2 poles (40.2897, 27.6738) (40.5081, 27.6738) (40.9449, 27.5717) (41.1661, 27.461) knots 0 0 0 1 2 2 2
  line L200 (41.1661, 27.461) -> (41.1661, 26.7576)
  line L201 (41.1661, 26.7576) -> (41.0611, 26.7576)
  spline S174 degree 2 poles (41.0611, 26.7576) (41.0101, 26.8059) (40.8683, 26.9193) (40.7832, 26.9647) knots 0 0 0 1 2 2 2
  spline S175 degree 2 poles (40.7832, 26.9647) (40.6924, 27.0157) (40.4684, 27.0838) (40.3294, 27.0838) knots 0 0 0 1 2 2 2
  spline S176 degree 2 poles (40.3294, 27.0838) (40.0145, 27.0838) (39.6685, 26.6442) (39.6685, 26.2698) knots 0 0 0 1 2 2 2
  spline S177 degree 2 poles (39.6685, 26.2698) (39.6685, 25.8727) (40.0372, 25.4813) (40.3436, 25.4813) knots 0 0 0 1 2 2 2
  spline S178 degree 2 poles (40.3436, 25.4813) (40.4996, 25.4813) (40.7321, 25.5522) (40.8172, 25.6033) knots 0 0 0 1 2 2 2
  spline S179 degree 2 poles (40.8172, 25.6033) (40.8995, 25.6515) (41.0186, 25.7593) (41.0611, 25.8018) knots 0 0 0 1 2 2 2
  line L202 (41.0611, 25.8018) -> (41.1661, 25.8018)
  line L203 (41.1661, 25.8018) -> (41.1661, 25.0956)
  spline S180 degree 2 poles (41.1661, 25.0956) (41.0952, 25.0644) (40.9108, 24.985) (40.8144, 24.9594) knots 0 0 0 1 2 2 2
  spline S181 degree 2 poles (40.8144, 24.9594) (40.6953, 24.9254) (40.4854, 24.8914) (40.3124, 24.8914) knots 0 0 0 1 2 2 2
  spline S182 degree 2 poles (44.0903, 26.2811) (44.0903, 25.6288) (43.3784, 24.88) (42.7289, 24.88) knots 0 0 0 1 2 2 2
  spline S183 degree 2 poles (42.7289, 24.88) (42.0822, 24.88) (41.3646, 25.6288) (41.3646, 26.2811) knots 0 0 0 1 2 2 2
  spline S184 degree 2 poles (41.3646, 26.2811) (41.3646, 26.9392) (42.0822, 27.6851) (42.7289, 27.6851) knots 0 0 0 1 2 2 2
  spline S185 degree 2 poles (42.7289, 27.6851) (43.3756, 27.6851) (44.0903, 26.9363) (44.0903, 26.2811) knots 0 0 0 1 2 2 2
  spline S186 degree 2 poles (43.2479, 26.2755) (43.2479, 26.5109) (43.1714, 26.8257) (43.1033, 26.9193) knots 0 0 0 1 2 2 2
  spline S187 degree 2 poles (43.1033, 26.9193) (43.0295, 27.0186) (42.8452, 27.0952) (42.7289, 27.0952) knots 0 0 0 1 2 2 2
  spline S188 degree 2 poles (42.7289, 27.0952) (42.6154, 27.0952) (42.4368, 27.0271) (42.363, 26.9307) knots 0 0 0 1 2 2 2
  spline S189 degree 2 poles (42.363, 26.9307) (42.2921, 26.8399) (42.207, 26.5194) (42.207, 26.2755) knots 0 0 0 1 2 2 2
  spline S190 degree 2 poles (42.207, 26.2755) (42.207, 26.0344) (42.2864, 25.7366) (42.3517, 25.6458) knots 0 0 0 1 2 2 2
  spline S191 degree 2 poles (42.3517, 25.6458) (42.4169, 25.555) (42.6154, 25.47) (42.7346, 25.47) knots 0 0 0 1 2 2 2
  spline S192 degree 2 poles (42.7346, 25.47) (42.8338, 25.47) (43.038, 25.555) (43.1004, 25.6401) knots 0 0 0 1 2 2 2
  spline S193 degree 2 poles (43.1004, 25.6401) (43.1714, 25.7394) (43.2479, 26.0259) (43.2479, 26.2755) knots 0 0 0 1 2 2 2
  line L204 (47.6782, 24.9623) -> (47.6782, 26.2811)
  spline S194 degree 2 poles (47.6782, 26.2811) (47.6782, 26.4768) (47.6641, 26.7435) (47.63, 26.8286) knots 0 0 0 1 2 2 2
  spline S195 degree 2 poles (47.63, 26.8286) (47.5932, 26.9136) (47.4457, 26.9902) (47.3124, 26.9902) knots 0 0 0 1 2 2 2
  spline S196 degree 2 poles (47.3124, 26.9902) (47.2188, 26.9902) (47.0372, 26.908) (46.9295, 26.8314) knots 0 0 0 1 2 2 2
  line L205 (46.9295, 26.8314) -> (46.9295, 24.9623)
  line L206 (46.9295, 24.9623) -> (46.1013, 24.9623)
  line L207 (46.1013, 24.9623) -> (46.1013, 26.2811)
  spline S197 degree 2 poles (46.1013, 26.2811) (46.1013, 26.474) (46.0842, 26.7435) (46.0502, 26.8286) knots 0 0 0 1 2 2 2
  spline S198 degree 2 poles (46.0502, 26.8286) (46.0133, 26.9136) (45.8658, 26.9902) (45.7325, 26.9902) knots 0 0 0 1 2 2 2
  spline S199 degree 2 poles (45.7325, 26.9902) (45.6333, 26.9902) (45.4376, 26.8966) (45.3468, 26.8314) knots 0 0 0 1 2 2 2
  line L208 (45.3468, 26.8314) -> (45.3468, 24.9623)
  line L209 (45.3468, 24.9623) -> (44.5243, 24.9623)
  line L210 (44.5243, 24.9623) -> (44.5243, 27.6029)
  line L211 (44.5243, 27.6029) -> (45.3468, 27.6029)
  line L212 (45.3468, 27.6029) -> (45.3468, 27.3107)
  spline S200 degree 2 poles (45.3468, 27.3107) (45.5482, 27.4809) (45.9084, 27.6738) (46.1325, 27.6738) knots 0 0 0 1 2 2 2
  spline S201 degree 2 poles (46.1325, 27.6738) (46.3735, 27.6738) (46.7423, 27.444) (46.8387, 27.2143) knots 0 0 0 1 2 2 2
  spline S202 degree 2 poles (46.8387, 27.2143) (47.0741, 27.4355) (47.4939, 27.6738) (47.7094, 27.6738) knots 0 0 0 1 2 2 2
  spline S203 degree 2 poles (47.7094, 27.6738) (47.8938, 27.6738) (48.1859, 27.5575) (48.2852, 27.4384) knots 0 0 0 1 2 2 2
  spline S204 degree 2 poles (48.2852, 27.4384) (48.3958, 27.3107) (48.5064, 26.9619) (48.5064, 26.6811) knots 0 0 0 1 2 2 2
  line L213 (48.5064, 26.6811) -> (48.5064, 24.9623)
  line L214 (48.5064, 24.9623) -> (47.6782, 24.9623)
  line L215 (51.147, 28.6183) -> (49.7544, 24.2021)
  line L216 (49.7544, 24.2021) -> (49.0794, 24.2021)
  line L217 (49.0794, 24.2021) -> (50.4692, 28.6183)
  line L218 (50.4692, 28.6183) -> (51.147, 28.6183)
  spline S205 degree 2 poles (54.2925, 25.2657) (54.2925, 24.8999) (54.0798, 24.3865) (53.8983, 24.2447) knots 0 0 0 1 2 2 2
  spline S206 degree 2 poles (53.8983, 24.2447) (53.7139, 24.1) (53.2034, 23.9696) (52.8914, 23.9696) knots 0 0 0 1 2 2 2
  spline S207 degree 2 poles (52.8914, 23.9696) (52.6276, 23.9696) (52.1539, 24.0376) (51.9809, 24.083) knots 0 0 0 1 2 2 2
  line L219 (51.9809, 24.083) -> (51.9809, 24.7439)
  line L220 (51.9809, 24.7439) -> (52.0774, 24.7439)
  spline S208 degree 2 poles (52.0774, 24.7439) (52.1369, 24.7212) (52.3043, 24.6644) (52.3893, 24.6418) knots 0 0 0 1 2 2 2
  spline S209 degree 2 poles (52.3893, 24.6418) (52.4915, 24.6162) (52.6843, 24.5822) (52.7836, 24.5822) knots 0 0 0 1 2 2 2
  spline S210 degree 2 poles (52.7836, 24.5822) (52.9935, 24.5822) (53.2714, 24.6673) (53.3423, 24.7467) knots 0 0 0 1 2 2 2
  spline S211 degree 2 poles (53.3423, 24.7467) (53.4133, 24.829) (53.47, 25.0502) (53.47, 25.2204) knots 0 0 0 1 2 2 2
  line L221 (53.47, 25.2204) -> (53.47, 25.2686)
  spline S212 degree 2 poles (53.47, 25.2686) (53.331, 25.1466) (52.968, 24.9991) (52.7751, 24.9991) knots 0 0 0 1 2 2 2
  spline S213 degree 2 poles (52.7751, 24.9991) (52.2617, 24.9991) (51.7058, 25.6657) (51.7058, 26.3492) knots 0 0 0 1 2 2 2
  spline S214 degree 2 poles (51.7058, 26.3492) (51.7058, 26.6584) (51.876, 27.1519) (52.0291, 27.3249) knots 0 0 0 1 2 2 2
  spline S215 degree 2 poles (52.0291, 27.3249) (52.1766, 27.4922) (52.5879, 27.6738) (52.812, 27.6738) knots 0 0 0 1 2 2 2
  spline S216 degree 2 poles (52.812, 27.6738) (53.0133, 27.6738) (53.3338, 27.5717) (53.4643, 27.4866) knots 0 0 0 1 2 2 2
  line L222 (53.4643, 27.4866) -> (53.4955, 27.6029)
  line L223 (53.4955, 27.6029) -> (54.2925, 27.6029)
  line L224 (54.2925, 27.6029) -> (54.2925, 25.2657)
  line L225 (53.47, 25.7933) -> (53.47, 26.9902)
  spline S217 degree 2 poles (53.47, 26.9902) (53.4104, 27.0186) (53.2317, 27.0555) (53.141, 27.0555) knots 0 0 0 1 2 2 2
  spline S218 degree 2 poles (53.141, 27.0555) (52.846, 27.0555) (52.5482, 26.6726) (52.5482, 26.3294) knots 0 0 0 1 2 2 2
  spline S219 degree 2 poles (52.5482, 26.3294) (52.5482, 26.1592) (52.5936, 25.9209) (52.6531, 25.8302) knots 0 0 0 1 2 2 2
  spline S220 degree 2 poles (52.6531, 25.8302) (52.7127, 25.7394) (52.9027, 25.6486) (53.0502, 25.6486) knots 0 0 0 1 2 2 2
  spline S221 degree 2 poles (53.0502, 25.6486) (53.1608, 25.6486) (53.3735, 25.7252) (53.47, 25.7933) knots 0 0 0 1 2 2 2
  spline S222 degree 2 poles (57.3217, 25.2657) (57.3217, 24.8999) (57.109, 24.3865) (56.9274, 24.2447) knots 0 0 0 1 2 2 2
  spline S223 degree 2 poles (56.9274, 24.2447) (56.7431, 24.1) (56.2325, 23.9696) (55.9205, 23.9696) knots 0 0 0 1 2 2 2
  spline S224 degree 2 poles (55.9205, 23.9696) (55.6568, 23.9696) (55.1831, 24.0376) (55.0101, 24.083) knots 0 0 0 1 2 2 2
  line L226 (55.0101, 24.083) -> (55.0101, 24.7439)
  line L227 (55.0101, 24.7439) -> (55.1065, 24.7439)
  spline S225 degree 2 poles (55.1065, 24.7439) (55.1661, 24.7212) (55.3334, 24.6644) (55.4185, 24.6418) knots 0 0 0 1 2 2 2
  spline S226 degree 2 poles (55.4185, 24.6418) (55.5206, 24.6162) (55.7135, 24.5822) (55.8128, 24.5822) knots 0 0 0 1 2 2 2
  spline S227 degree 2 poles (55.8128, 24.5822) (56.0227, 24.5822) (56.3006, 24.6673) (56.3715, 24.7467) knots 0 0 0 1 2 2 2
  spline S228 degree 2 poles (56.3715, 24.7467) (56.4424, 24.829) (56.4992, 25.0502) (56.4992, 25.2204) knots 0 0 0 1 2 2 2
  line L228 (56.4992, 25.2204) -> (56.4992, 25.2686)
  spline S229 degree 2 poles (56.4992, 25.2686) (56.3602, 25.1466) (55.9971, 24.9991) (55.8043, 24.9991) knots 0 0 0 1 2 2 2
  spline S230 degree 2 poles (55.8043, 24.9991) (55.2909, 24.9991) (54.735, 25.6657) (54.735, 26.3492) knots 0 0 0 1 2 2 2
  spline S231 degree 2 poles (54.735, 26.3492) (54.735, 26.6584) (54.9051, 27.1519) (55.0583, 27.3249) knots 0 0 0 1 2 2 2
  spline S232 degree 2 poles (55.0583, 27.3249) (55.2058, 27.4922) (55.6171, 27.6738) (55.8411, 27.6738) knots 0 0 0 1 2 2 2
  spline S233 degree 2 poles (55.8411, 27.6738) (56.0425, 27.6738) (56.363, 27.5717) (56.4935, 27.4866) knots 0 0 0 1 2 2 2
  line L229 (56.4935, 27.4866) -> (56.5247, 27.6029)
  line L230 (56.5247, 27.6029) -> (57.3217, 27.6029)
  line L231 (57.3217, 27.6029) -> (57.3217, 25.2657)
  line L232 (56.4992, 25.7933) -> (56.4992, 26.9902)
  spline S234 degree 2 poles (56.4992, 26.9902) (56.4396, 27.0186) (56.2609, 27.0555) (56.1701, 27.0555) knots 0 0 0 1 2 2 2
  spline S235 degree 2 poles (56.1701, 27.0555) (55.8752, 27.0555) (55.5774, 26.6726) (55.5774, 26.3294) knots 0 0 0 1 2 2 2
  spline S236 degree 2 poles (55.5774, 26.3294) (55.5774, 26.1592) (55.6227, 25.9209) (55.6823, 25.8302) knots 0 0 0 1 2 2 2
  spline S237 degree 2 poles (55.6823, 25.8302) (55.7419, 25.7394) (55.9319, 25.6486) (56.0794, 25.6486) knots 0 0 0 1 2 2 2
  spline S238 degree 2 poles (56.0794, 25.6486) (56.19, 25.6486) (56.4027, 25.7252) (56.4992, 25.7933) knots 0 0 0 1 2 2 2
  spline S239 degree 2 poles (60.5551, 25.9351) (60.5551, 25.711) (60.3679, 25.3225) (60.1892, 25.1807) knots 0 0 0 1 2 2 2
  spline S240 degree 2 poles (60.1892, 25.1807) (60.0105, 25.0388) (59.4971, 24.88) (59.1653, 24.88) knots 0 0 0 1 2 2 2
  spline S241 degree 2 poles (59.1653, 24.88) (58.8107, 24.88) (58.2804, 25.0417) (58.1102, 25.1807) knots 0 0 0 1 2 2 2
  spline S242 degree 2 poles (58.1102, 25.1807) (57.9428, 25.3196) (57.784, 25.6969) (57.784, 25.9068) knots 0 0 0 1 2 2 2
  spline S243 degree 2 poles (57.784, 25.9068) (57.784, 26.2074) (58.1158, 26.6073) (58.4307, 26.7406) knots 0 0 0 1 2 2 2
  line L233 (58.4307, 26.7406) -> (58.4307, 26.7548)
  spline S244 degree 2 poles (58.4307, 26.7548) (58.1215, 26.9051) (57.8776, 27.3334) (57.8776, 27.5972) knots 0 0 0 1 2 2 2
  spline S245 degree 2 poles (57.8776, 27.5972) (57.8776, 27.7901) (58.0478, 28.1276) (58.2151, 28.2609) knots 0 0 0 1 2 2 2
  spline S246 degree 2 poles (58.2151, 28.2609) (58.3768, 28.3885) (58.8675, 28.5417) (59.1738, 28.5417) knots 0 0 0 1 2 2 2
  spline S247 degree 2 poles (59.1738, 28.5417) (59.4971, 28.5417) (59.9793, 28.4027) (60.1353, 28.2892) knots 0 0 0 1 2 2 2
  spline S248 degree 2 poles (60.1353, 28.2892) (60.2941, 28.1758) (60.4643, 27.8468) (60.4643, 27.6568) knots 0 0 0 1 2 2 2
  spline S249 degree 2 poles (60.4643, 27.6568) (60.4643, 27.4072) (60.175, 27.0072) (59.8772, 26.8683) knots 0 0 0 1 2 2 2
  line L234 (59.8772, 26.8683) -> (59.8772, 26.8569)
  spline S250 degree 2 poles (59.8772, 26.8569) (60.2261, 26.7151) (60.5551, 26.2556) (60.5551, 25.9351) knots 0 0 0 1 2 2 2
  spline S251 degree 2 poles (59.6872, 25.8982) (59.6872, 26.0713) (59.5397, 26.2528) (59.3014, 26.3691) knots 0 0 0 1 2 2 2
  spline S252 degree 2 poles (59.3014, 26.3691) (59.2333, 26.4003) (58.9752, 26.4995) (58.876, 26.5421) knots 0 0 0 1 2 2 2
  spline S253 degree 2 poles (58.876, 26.5421) (58.7852, 26.4513) (58.6406, 26.179) (58.6406, 26.0174) knots 0 0 0 1 2 2 2
  spline S254 degree 2 poles (58.6406, 26.0174) (58.6406, 25.7734) (58.9526, 25.4813) (59.205, 25.4813) knots 0 0 0 1 2 2 2
  spline S255 degree 2 poles (59.205, 25.4813) (59.2759, 25.4813) (59.4517, 25.5267) (59.5198, 25.5721) knots 0 0 0 1 2 2 2
  spline S256 degree 2 poles (59.5198, 25.5721) (59.5964, 25.626) (59.6872, 25.7734) (59.6872, 25.8982) knots 0 0 0 1 2 2 2
  spline S257 degree 2 poles (59.6106, 27.5546) (59.6106, 27.7333) (59.3752, 27.9461) (59.1738, 27.9461) knots 0 0 0 1 2 2 2
  spline S258 degree 2 poles (59.1738, 27.9461) (58.9809, 27.9461) (58.7455, 27.7532) (58.7455, 27.6114) knots 0 0 0 1 2 2 2
  spline S259 degree 2 poles (58.7455, 27.6114) (58.7455, 27.4724) (58.8873, 27.2994) (59.0376, 27.2285) knots 0 0 0 1 2 2 2
  spline S260 degree 2 poles (59.0376, 27.2285) (59.1029, 27.1944) (59.2844, 27.1235) (59.4347, 27.0668) knots 0 0 0 1 2 2 2
  spline S261 degree 2 poles (59.4347, 27.0668) (59.5255, 27.1859) (59.6106, 27.41) (59.6106, 27.5546) knots 0 0 0 1 2 2 2
  spline S262 degree 2 poles (63.6211, 25.9351) (63.6211, 25.711) (63.4339, 25.3225) (63.2552, 25.1807) knots 0 0 0 1 2 2 2
  spline S263 degree 2 poles (63.2552, 25.1807) (63.0765, 25.0388) (62.5632, 24.88) (62.2313, 24.88) knots 0 0 0 1 2 2 2
  spline S264 degree 2 poles (62.2313, 24.88) (61.8768, 24.88) (61.3464, 25.0417) (61.1762, 25.1807) knots 0 0 0 1 2 2 2
  spline S265 degree 2 poles (61.1762, 25.1807) (61.0089, 25.3196) (60.85, 25.6969) (60.85, 25.9068) knots 0 0 0 1 2 2 2
  spline S266 degree 2 poles (60.85, 25.9068) (60.85, 26.2074) (61.1819, 26.6073) (61.4967, 26.7406) knots 0 0 0 1 2 2 2
  line L235 (61.4967, 26.7406) -> (61.4967, 26.7548)
  spline S267 degree 2 poles (61.4967, 26.7548) (61.1876, 26.9051) (60.9436, 27.3334) (60.9436, 27.5972) knots 0 0 0 1 2 2 2
  spline S268 degree 2 poles (60.9436, 27.5972) (60.9436, 27.7901) (61.1138, 28.1276) (61.2812, 28.2609) knots 0 0 0 1 2 2 2
  spline S269 degree 2 poles (61.2812, 28.2609) (61.4428, 28.3885) (61.9335, 28.5417) (62.2398, 28.5417) knots 0 0 0 1 2 2 2
  spline S270 degree 2 poles (62.2398, 28.5417) (62.5632, 28.5417) (63.0453, 28.4027) (63.2013, 28.2892) knots 0 0 0 1 2 2 2
  spline S271 degree 2 poles (63.2013, 28.2892) (63.3602, 28.1758) (63.5304, 27.8468) (63.5304, 27.6568) knots 0 0 0 1 2 2 2
  spline S272 degree 2 poles (63.5304, 27.6568) (63.5304, 27.4072) (63.241, 27.0072) (62.9432, 26.8683) knots 0 0 0 1 2 2 2
  line L236 (62.9432, 26.8683) -> (62.9432, 26.8569)
  spline S273 degree 2 poles (62.9432, 26.8569) (63.2921, 26.7151) (63.6211, 26.2556) (63.6211, 25.9351) knots 0 0 0 1 2 2 2
  spline S274 degree 2 poles (62.7532, 25.8982) (62.7532, 26.0713) (62.6057, 26.2528) (62.3675, 26.3691) knots 0 0 0 1 2 2 2
  spline S275 degree 2 poles (62.3675, 26.3691) (62.2994, 26.4003) (62.0413, 26.4995) (61.942, 26.5421) knots 0 0 0 1 2 2 2
  spline S276 degree 2 poles (61.942, 26.5421) (61.8513, 26.4513) (61.7066, 26.179) (61.7066, 26.0174) knots 0 0 0 1 2 2 2
  spline S277 degree 2 poles (61.7066, 26.0174) (61.7066, 25.7734) (62.0186, 25.4813) (62.271, 25.4813) knots 0 0 0 1 2 2 2
  spline S278 degree 2 poles (62.271, 25.4813) (62.3419, 25.4813) (62.5178, 25.5267) (62.5859, 25.5721) knots 0 0 0 1 2 2 2
  spline S279 degree 2 poles (62.5859, 25.5721) (62.6624, 25.626) (62.7532, 25.7734) (62.7532, 25.8982) knots 0 0 0 1 2 2 2
  spline S280 degree 2 poles (62.6766, 27.5546) (62.6766, 27.7333) (62.4412, 27.9461) (62.2398, 27.9461) knots 0 0 0 1 2 2 2
  spline S281 degree 2 poles (62.2398, 27.9461) (62.047, 27.9461) (61.8116, 27.7532) (61.8116, 27.6114) knots 0 0 0 1 2 2 2
  spline S282 degree 2 poles (61.8116, 27.6114) (61.8116, 27.4724) (61.9534, 27.2994) (62.1037, 27.2285) knots 0 0 0 1 2 2 2
  spline S283 degree 2 poles (62.1037, 27.2285) (62.1689, 27.1944) (62.3504, 27.1235) (62.5008, 27.0668) knots 0 0 0 1 2 2 2
  spline S284 degree 2 poles (62.5008, 27.0668) (62.5915, 27.1859) (62.6766, 27.41) (62.6766, 27.5546) knots 0 0 0 1 2 2 2
  line L237 (66.5397, 24.9623) -> (64.2281, 24.9623)
  line L238 (64.2281, 24.9623) -> (64.2281, 25.5721)
  line L239 (64.2281, 25.5721) -> (64.9655, 25.5721)
  line L240 (64.9655, 25.5721) -> (64.9655, 27.4242)
  line L241 (64.9655, 27.4242) -> (64.2281, 27.4242)
  line L242 (64.2281, 27.4242) -> (64.2281, 27.9943)